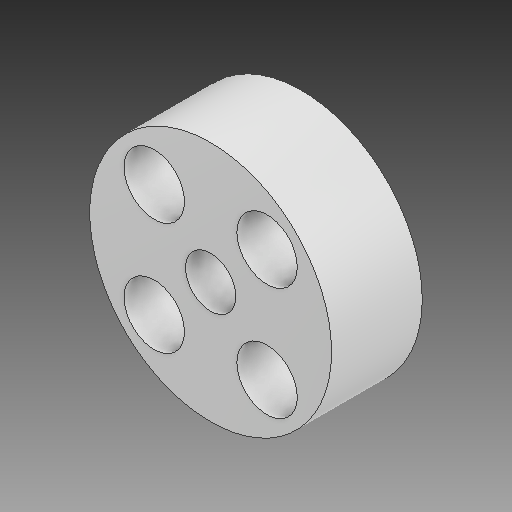
# Autodesk Inventor part: 脚最終段カム3
Saved by Autodesk Inventor 2020 (Build 240168000, 168)
## iProperties
Created: 2019-07-24
Part Number: 脚最終段カム3
Material: アルミニウム 2014-T4
Document SubType Name: Modeling
Designer: 雪村
Density: 2.8 g/cm^3
Appearance: サテン
Mass: 1.00692 g
Surface Area: 5.34463 cm^2
Volume: 0.359614 cm^3
Description: アルミ7000 5t(4.5t)
Author: 雪村
Autodesk Inventor part; units mm, degrees
ref_plane "YZ Plane" through (0, 0, 0) normal (1, 0, 0) x (0, 1, 0)
ref_plane "XZ Plane" through (0, 0, 0) normal (0, 1, 0) x (-1, 0, 0)
ref_plane "XY Plane" through (0, 0, 0) normal (0, 0, 1) x (1, 0, 0)
sketch "スケッチ1" plane through (0, 0, 0) normal (0, 0, 1) x (1, 0, 0)
  line L0 (-2.8, 2.8) -> (2.8, 2.8) construction
  line L1 (2.8, 2.8) -> (2.8, -2.8) construction
  line L2 (2.8, -2.8) -> (-2.8, -2.8) construction
  line L3 (-2.8, -2.8) -> (-2.8, 2.8) construction
  circle A0 centre (-2.8, 2.8) radius 1.5
  circle A1 centre (2.8, 2.8) radius 1.5
  circle A2 centre (2.8, -2.8) radius 1.5
  circle A3 centre (-2.8, -2.8) radius 1.5
  circle A4 centre (0, 0) radius 1.25
  circle A5 centre (0, 0) radius 6
  dimension "d0" = 3
  dimension "d1" = 3
  dimension "d2" = 3
  dimension "d3" = 3
  dimension "d4" = 5.6
  dimension "d5" = 2.5
  dimension "d6" = 12
  constraints: 8 end point, 7 coincident, 6 centre point, 1 horizontal, 9 other
  measures "d0" diameter of A0
  measures "d1" diameter of A1
  measures "d2" diameter of A2
  measures "d3" diameter of A3
  measures "d4" distance of L0.start L0.end
  measures "d5" diameter of A4
  measures "d6" diameter of A5
extrude "押し出し1" add sketch "スケッチ1" along normal blind 4.5
